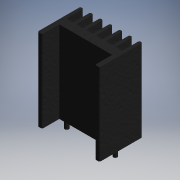
# Autodesk Inventor part: WA-T247-101E
Saved by Autodesk Inventor 2018.3 (Build 223284000, 284)
## iProperties
Part Number: WA-T247-101E
Material: Generic
Document SubType Name: Modeling
Designer: Gregor Gombač
Mass: 4.51501 g
Surface Area: 52.4888 cm^2
Volume: 4.51501 cm^3
Density: 1 g/cm^3
Appearance: Black
Title: 247
Author: SYSTEM
Revision Number: 5LAST_VERSION
Sending System: PRO/ENGINEER BY PARAMETRIC TECHNOLOGY CORPORATION, 2016360
Preprocessor: PRO/ENGINEER BY PARAMETRIC TECHNOLOGY CORPORATION, 2016360
Autodesk Inventor part; units mm, degrees
ref_plane "YZ Plane" through (0, 0, 0) normal (1, 0, 0) x (0, 1, 0)
ref_plane "XZ Plane" through (0, 0, 0) normal (0, 1, 0) x (-1, 0, 0)
ref_plane "Work Plane1" through (-9.8235, 15.24, 1.6002) normal (0, 1, 0) x (1, 0, 0)
sketch "Sketch1" plane through (-9.8235, 15.24, 1.6002) normal (0, 1, 0) x (1, 0, 0)
  line L0 (-1.2255, -6.4008) -> (-0.508, -6.4008)
  arc A0 (-1.7335, -5.8928) -> (-1.2255, -6.4008) centre (-1.2255, -5.8928) ccw
  line L1 (-1.7335, 9.0932) -> (-1.7335, -5.8928)
  arc A1 (-0.508, -6.4008) -> (0, -5.8928) centre (-0.508, -5.8928) ccw
  line L2 (0, -5.8928) -> (0, 0)
  line L3 (-1.0858, 9.6012) -> (-1.2256, 9.6012)
  arc A2 (-0.5778, 9.0932) -> (-1.0858, 9.6012) centre (-1.0858, 9.0932) ccw
  line L4 (0, 0) -> (19.6469, 0)
  line L5 (19.6469, 0) -> (19.6469, -5.8928)
  arc A3 (19.6469, -5.8928) -> (20.1549, -6.4008) centre (20.1549, -5.8928) ccw
  line L6 (20.1549, -6.4008) -> (20.8725, -6.4008)
  arc A4 (20.8725, -6.4008) -> (21.3804, -5.8928) centre (20.8725, -5.8928) ccw
  line L7 (21.3804, -5.8928) -> (21.3804, 9.0932)
  arc A5 (21.3804, 9.0932) -> (20.8725, 9.6012) centre (20.8725, 9.0932) ccw
  arc A6 (20.7327, 9.6012) -> (20.2247, 9.0932) centre (20.7327, 9.0932) ccw
  line L8 (20.8725, 9.6012) -> (20.7327, 9.6012)
  line L9 (-0.5778, 9.0932) -> (-0.5778, 3.7084)
  arc A7 (-0.5778, 3.7084) -> (-0.0698, 3.2004) centre (-0.0698, 3.7084) ccw
  line L10 (-0.0698, 3.2004) -> (1.4182, 3.2004)
  arc A8 (1.4182, 3.2004) -> (1.9262, 3.7084) centre (1.4182, 3.7084) ccw
  line L11 (1.9262, 3.7084) -> (1.9262, 9.0932)
  arc A9 (-0.5778, 9.0932) -> (-1.0858, 9.6012) centre (-1.0859, 9.0932) ccw
  arc A10 (-1.2256, 9.6012) -> (-1.7335, 9.0932) centre (-1.2256, 9.0932) ccw
  line L12 (-1.2256, 9.6012) -> (-1.0858, 9.6012)
  arc A11 (2.4342, 9.6012) -> (1.9262, 9.0932) centre (2.4342, 9.0932) ccw
  line L13 (2.4342, 9.6012) -> (2.5739, 9.6012)
  arc A12 (3.0819, 9.0932) -> (2.5739, 9.6012) centre (2.5739, 9.0932) ccw
  line L14 (3.0819, 9.0932) -> (3.0819, 3.7084)
  arc A13 (3.0819, 3.7084) -> (3.5899, 3.2004) centre (3.5899, 3.7084) ccw
  line L15 (3.5899, 3.2004) -> (5.0779, 3.2004)
  arc A14 (5.0779, 3.2004) -> (5.5859, 3.7084) centre (5.0779, 3.7084) ccw
  line L16 (5.5859, 3.7084) -> (5.5859, 9.0932)
  arc A15 (6.0939, 9.6012) -> (5.5859, 9.0932) centre (6.0939, 9.0932) ccw
  line L17 (6.0939, 9.6012) -> (6.2336, 9.6012)
  arc A16 (6.7416, 9.0932) -> (6.2336, 9.6012) centre (6.2336, 9.0932) ccw
  line L18 (6.7416, 9.0932) -> (6.7416, 3.7084)
  arc A17 (6.7416, 3.7084) -> (7.2496, 3.2004) centre (7.2496, 3.7084) ccw
  line L19 (7.2496, 3.2004) -> (8.7376, 3.2004)
  arc A18 (8.7376, 3.2004) -> (9.2456, 3.7084) centre (8.7376, 3.7084) ccw
  line L20 (9.2456, 3.7084) -> (9.2456, 9.0932)
  arc A19 (9.7536, 9.6012) -> (9.2456, 9.0932) centre (9.7536, 9.0932) ccw
  line L21 (9.7536, 9.6012) -> (9.8933, 9.6012)
  arc A20 (10.4013, 9.0932) -> (9.8933, 9.6012) centre (9.8933, 9.0932) ccw
  line L22 (10.4013, 9.0932) -> (10.4013, 3.7084)
  arc A21 (10.4013, 3.7084) -> (10.9093, 3.2004) centre (10.9093, 3.7084) ccw
  line L23 (10.9093, 3.2004) -> (12.3973, 3.2004)
  arc A22 (12.3973, 3.2004) -> (12.9053, 3.7084) centre (12.3973, 3.7084) ccw
  line L24 (12.9053, 3.7084) -> (12.9053, 9.0932)
  arc A23 (13.4133, 9.6012) -> (12.9053, 9.0932) centre (13.4133, 9.0932) ccw
  line L25 (13.4133, 9.6012) -> (13.553, 9.6012)
  arc A24 (14.061, 9.0932) -> (13.553, 9.6012) centre (13.553, 9.0932) ccw
  line L26 (14.061, 9.0932) -> (14.061, 3.7084)
  arc A25 (14.061, 3.7084) -> (14.569, 3.2004) centre (14.569, 3.7084) ccw
  line L27 (14.569, 3.2004) -> (16.057, 3.2004)
  arc A26 (16.057, 3.2004) -> (16.565, 3.7084) centre (16.057, 3.7084) ccw
  line L28 (16.565, 3.7084) -> (16.565, 9.0932)
  arc A27 (17.073, 9.6012) -> (16.565, 9.0932) centre (17.073, 9.0932) ccw
  line L29 (17.073, 9.6012) -> (17.2127, 9.6012)
  arc A28 (17.7207, 9.0932) -> (17.2127, 9.6012) centre (17.2127, 9.0932) ccw
  line L30 (17.7207, 9.0932) -> (17.7207, 3.7084)
  arc A29 (17.7207, 3.7084) -> (18.2287, 3.2004) centre (18.2287, 3.7084) ccw
  line L31 (18.2287, 3.2004) -> (19.7167, 3.2004)
  arc A30 (19.7167, 3.2004) -> (20.2247, 3.7084) centre (19.7167, 3.7084) ccw
  line L32 (20.2247, 3.7084) -> (20.2247, 9.0932)
  dimension "d0" = 21.9583
  dimension "d1" = 3.6597
  constraints: 66 end point, 62 point on circle, 31 centre point, 16 horizontal, 16 vertical, 9 tangent, 1 collinear, 1 equal radius, 1 parallel, 1 perpendicular, 28 other
  measures "d0" distance of L32.end L1.start
  measures "d1" distance of L11.end L1.start
sketch "Sketch2" plane through (0, 0, 0) normal (0, 1, 0) x (-1, 0, 0)
  line L0 (-9.8235, 1.6002) -> (-9.8235, 7.493) projected
  arc A0 (-9.8235, 7.493) -> (-10.3314, 8.001) centre (-10.3314, 7.493) ccw projected
  line L1 (-10.3314, 8.001) -> (-11.049, 8.001) projected
  arc A1 (-11.049, 8.001) -> (-11.557, 7.493) centre (-11.049, 7.493) ccw projected
  line L2 (-11.557, 7.493) -> (-11.557, -7.493) projected
  arc A2 (-11.557, -7.493) -> (-11.049, -8.001) centre (-11.049, -7.493) ccw projected
  arc A3 (-10.9093, -8.001) -> (-10.4013, -7.493) centre (-10.9093, -7.493) ccw projected
  line L3 (-10.4013, -2.1082) -> (-10.4013, -7.493) projected
  arc A4 (-9.8933, -1.6002) -> (-10.4013, -2.1082) centre (-9.8933, -2.1082) ccw projected
  line L4 (-8.4053, -1.6002) -> (-9.8933, -1.6002) projected
  line L5 (-11.049, -8.001) -> (-10.9093, -8.001) projected
  arc A5 (-7.8973, -2.1082) -> (-8.4053, -1.6002) centre (-8.4053, -2.1082) ccw projected
  line L6 (-7.8973, -7.493) -> (-7.8973, -2.1082) projected
  arc A6 (-7.8973, -7.493) -> (-7.3893, -8.001) centre (-7.3893, -7.493) ccw projected
  line L7 (-7.2496, -8.001) -> (-7.3893, -8.001) projected
  arc A7 (-7.2496, -8.001) -> (-6.7416, -7.493) centre (-7.2496, -7.493) ccw projected
  line L8 (-6.7416, -2.1082) -> (-6.7416, -7.493) projected
  arc A8 (-6.2336, -1.6002) -> (-6.7416, -2.1082) centre (-6.2336, -2.1082) ccw projected
  line L9 (-4.7456, -1.6002) -> (-6.2336, -1.6002) projected
  arc A9 (-4.2376, -2.1082) -> (-4.7456, -1.6002) centre (-4.7456, -2.1082) ccw projected
  line L10 (-4.2376, -7.493) -> (-4.2376, -2.1082) projected
  arc A10 (-4.2376, -7.493) -> (-3.7296, -8.001) centre (-3.7296, -7.493) ccw projected
  line L11 (-3.5899, -8.001) -> (-3.7296, -8.001) projected
  arc A11 (-3.5899, -8.001) -> (-3.0819, -7.493) centre (-3.5899, -7.493) ccw projected
  line L12 (-3.0819, -2.1082) -> (-3.0819, -7.493) projected
  arc A12 (-2.5739, -1.6002) -> (-3.0819, -2.1082) centre (-2.5739, -2.1082) ccw projected
  line L13 (-1.0858, -1.6002) -> (-2.5739, -1.6002) projected
  arc A13 (-0.5778, -2.1082) -> (-1.0858, -1.6002) centre (-1.0858, -2.1082) ccw projected
  line L14 (-0.5778, -7.493) -> (-0.5778, -2.1082) projected
  arc A14 (-0.5778, -7.493) -> (-0.0698, -8.001) centre (-0.0698, -7.493) ccw projected
  line L15 (0.0699, -8.001) -> (-0.0698, -8.001) projected
  arc A15 (0.0699, -8.001) -> (0.5779, -7.493) centre (0.0699, -7.493) ccw projected
  line L16 (0.5779, -2.1082) -> (0.5779, -7.493) projected
  arc A16 (1.0859, -1.6002) -> (0.5779, -2.1082) centre (1.0859, -2.1082) ccw projected
  line L17 (2.5739, -1.6002) -> (1.0859, -1.6002) projected
  arc A17 (3.0819, -2.1082) -> (2.5739, -1.6002) centre (2.5739, -2.1082) ccw projected
  line L18 (3.0819, -7.493) -> (3.0819, -2.1082) projected
  arc A18 (3.0819, -7.493) -> (3.5899, -8.001) centre (3.5899, -7.493) ccw projected
  line L19 (3.7296, -8.001) -> (3.5899, -8.001) projected
  arc A19 (3.7296, -8.001) -> (4.2376, -7.493) centre (3.7296, -7.493) ccw projected
  line L20 (4.2376, -2.1082) -> (4.2376, -7.493) projected
  arc A20 (4.7456, -1.6002) -> (4.2376, -2.1082) centre (4.7456, -2.1082) ccw projected
  line L21 (6.2336, -1.6002) -> (4.7456, -1.6002) projected
  arc A21 (6.7416, -2.1082) -> (6.2336, -1.6002) centre (6.2336, -2.1082) ccw projected
  line L22 (6.7416, -7.493) -> (6.7416, -2.1082) projected
  arc A22 (6.7416, -7.493) -> (7.2496, -8.001) centre (7.2496, -7.493) ccw projected
  line L23 (7.3893, -8.001) -> (7.2496, -8.001) projected
  arc A23 (7.3893, -8.001) -> (7.8973, -7.493) centre (7.3893, -7.493) ccw projected
  line L24 (7.8973, -2.1082) -> (7.8973, -7.493) projected
  arc A24 (8.4053, -1.6002) -> (7.8973, -2.1082) centre (8.4053, -2.1082) ccw projected
  line L25 (9.8933, -1.6002) -> (8.4053, -1.6002) projected
  arc A25 (10.4013, -2.1082) -> (9.8933, -1.6002) centre (9.8933, -2.1082) ccw projected
  line L26 (10.4013, -7.493) -> (10.4013, -2.1082) projected
  arc A26 (10.4013, -7.493) -> (10.9093, -8.001) centre (10.9093, -7.493) ccw projected
  line L27 (10.9093, -8.001) -> (11.049, -8.001) projected
  arc A27 (11.049, -8.001) -> (11.557, -7.493) centre (11.049, -7.493) ccw projected
  line L28 (11.557, -7.493) -> (11.557, 7.493) projected
  arc A28 (11.557, 7.493) -> (11.049, 8.001) centre (11.049, 7.493) ccw projected
  line L29 (11.049, 8.001) -> (10.3315, 8.001) projected
  arc A29 (10.3315, 8.001) -> (9.8235, 7.493) centre (10.3315, 7.493) ccw projected
  line L30 (9.8235, 7.493) -> (9.8235, 1.6002) projected
  line L31 (9.8235, 1.6002) -> (-9.8235, 1.6002) projected
  point P0 (0, 0)
extrude "Extrusion1" add sketch "Sketch2" along normal blind 30.5
sketch "Sketch3" plane through (0, 0, 0) normal (0, -1, 0) x (1, 0, 0)
  line L0 (-9.8235, 1.6002) -> (9.8235, 1.6002) construction
  circle A0 centre (9.05, -0.3998) radius 0.75
  circle A1 centre (-9.05, -0.3998) radius 0.75
  line L1 (9.05, -0.3998) -> (0, 0) construction
  line L2 (0, 0) -> (-9.05, -0.3998) construction
  dimension "d11" = 1.5
  dimension "d12" = 2
  dimension "d13" = 18.1
  constraints: 4 end point, 2 centre point, 1 equal length, 1 equal radius, 1 horizontal alignment
  measures "d11" diameter of A0
  measures "d12" distance from line of L0 L1.start
  measures "d13" distance of L2.end L1.start
extrude "Extrusion2" add sketch "Sketch3" along normal blind 3.6
equation "\"d1\" = 0.166667 * d0"
body "Solid2"
